Autodesk Inventor part; units mm, degrees
(part 3 of 3)
sketch "LED Slots Sketch" plane through (-133.332, 2.75, -3) normal (0, 1, 0) x (1, 0, 0)
  line L0 (133.332, -3) -> (0, -3) construction
  line L1 (116.6655, -31.8672) -> (16.6665, -31.8672) construction
  line L2 (83.3325, -89.6017) -> (49.9995, -89.6017) construction
  line L3 (116.6655, -31.8672) -> (116.6655, -3) construction
  line L4 (99.999, -60.7344) -> (33.333, -60.7344) construction
  line L5 (99.999, -60.7344) -> (99.999, -31.8672) construction
  line L6 (83.3325, -89.6017) -> (83.3325, -60.7344) construction
  line L7 (66.666, -118.4689) -> (66.666, -89.6017) construction
  line L8 (49.9995, -89.6017) -> (49.9995, -3) construction
  line L9 (16.6665, -31.8672) -> (16.6665, -3) construction
  line L10 (33.333, -60.7344) -> (33.333, -3) construction
  line L11 (66.666, -89.6017) -> (66.666, -3) construction
  line L12 (83.3325, -60.7344) -> (83.3325, -3) construction
  line L13 (99.999, -31.8672) -> (99.999, -3) construction
  line L14 (102.499, -19.9336) -> (97.499, -19.9336) construction
  line L15 (97.499, -19.9336) -> (97.499, -14.9336) construction
  line L16 (97.499, -14.9336) -> (102.499, -14.9336) construction
  line L17 (102.499, -14.9336) -> (102.499, -19.9336) construction
  line L18 (99.999, -22.5586) -> (99.999, -12.3086) construction
  line L19 (108.3322, -17.4336) -> (91.6657, -17.4336) construction
  line L20 (96.999, -20.4336) -> (94.499, -20.4336) construction
  line L21 (94.499, -20.4336) -> (94.499, -14.4336) construction
  line L22 (94.499, -14.4336) -> (96.999, -14.4336) construction
  line L23 (96.999, -14.4336) -> (96.999, -20.4336) construction
  line L24 (108.3322, -22.5586) -> (91.6657, -22.5586) construction
  line L25 (91.6657, -22.5586) -> (91.6657, -12.3086) construction
  line L26 (91.6657, -12.3086) -> (108.3322, -12.3086) construction
  line L27 (108.3322, -12.3086) -> (108.3322, -22.5586) construction
  line L28 (104.499, -12.3086) -> (104.499, -22.5586) construction
  line L29 (92.499, -12.3086) -> (92.499, -22.5586) construction
  line L30 (85.8325, -19.9336) -> (80.8325, -19.9336) construction
  line L31 (80.8325, -19.9336) -> (80.8325, -14.9336) construction
  line L32 (80.8325, -14.9336) -> (85.8325, -14.9336) construction
  line L33 (85.8325, -14.9336) -> (85.8325, -19.9336) construction
  line L34 (83.3325, -22.5586) -> (83.3325, -12.3086) construction
  line L35 (91.6657, -17.4336) -> (74.9992, -17.4336) construction
  line L36 (80.3325, -20.4336) -> (77.8325, -20.4336) construction
  line L37 (77.8325, -20.4336) -> (77.8325, -14.4336) construction
  line L38 (77.8325, -14.4336) -> (80.3325, -14.4336) construction
  line L39 (80.3325, -14.4336) -> (80.3325, -20.4336) construction
  line L40 (91.6657, -22.5586) -> (74.9992, -22.5586) construction
  line L41 (74.9992, -22.5586) -> (74.9992, -12.3086) construction
  line L42 (74.9992, -12.3086) -> (91.6657, -12.3086) construction
  line L43 (91.6657, -12.3086) -> (91.6657, -22.5586) construction
  line L44 (87.8325, -12.3086) -> (87.8325, -22.5586) construction
  line L45 (75.8325, -12.3086) -> (75.8325, -22.5586) construction
  line L46 (69.166, -19.9336) -> (64.166, -19.9336) construction
  line L47 (64.166, -19.9336) -> (64.166, -14.9336) construction
  line L48 (64.166, -14.9336) -> (69.166, -14.9336) construction
  line L49 (69.166, -14.9336) -> (69.166, -19.9336) construction
  line L50 (66.666, -22.5586) -> (66.666, -12.3086) construction
  line L51 (74.9992, -17.4336) -> (58.3327, -17.4336) construction
  line L52 (63.666, -20.4336) -> (61.166, -20.4336) construction
  line L53 (61.166, -20.4336) -> (61.166, -14.4336) construction
  line L54 (61.166, -14.4336) -> (63.666, -14.4336) construction
  line L55 (63.666, -14.4336) -> (63.666, -20.4336) construction
  line L56 (74.9992, -22.5586) -> (58.3327, -22.5586) construction
  line L57 (58.3327, -22.5586) -> (58.3327, -12.3086) construction
  line L58 (58.3327, -12.3086) -> (74.9992, -12.3086) construction
  line L59 (74.9992, -12.3086) -> (74.9992, -22.5586) construction
  line L60 (71.166, -12.3086) -> (71.166, -22.5586) construction
  line L61 (59.166, -12.3086) -> (59.166, -22.5586) construction
  line L62 (35.833, -19.9336) -> (30.833, -19.9336) construction
  line L63 (30.833, -19.9336) -> (30.833, -14.9336) construction
  line L64 (30.833, -14.9336) -> (35.833, -14.9336) construction
  line L65 (35.833, -14.9336) -> (35.833, -19.9336) construction
  line L66 (33.333, -22.5586) -> (33.333, -12.3086) construction
  line L67 (41.6662, -17.4336) -> (24.9997, -17.4336) construction
  line L68 (30.333, -20.4336) -> (27.833, -20.4336) construction
  line L69 (27.833, -20.4336) -> (27.833, -14.4336) construction
  line L70 (27.833, -14.4336) -> (30.333, -14.4336) construction
  line L71 (30.333, -14.4336) -> (30.333, -20.4336) construction
  line L72 (41.6662, -22.5586) -> (24.9997, -22.5586) construction
  line L73 (24.9997, -22.5586) -> (24.9997, -12.3086) construction
  line L74 (24.9997, -12.3086) -> (41.6662, -12.3086) construction
  line L75 (41.6662, -12.3086) -> (41.6662, -22.5586) construction
  line L76 (37.833, -12.3086) -> (37.833, -22.5586) construction
  line L77 (25.833, -12.3086) -> (25.833, -22.5586) construction
  line L78 (52.4995, -19.9336) -> (47.4995, -19.9336) construction
  line L79 (47.4995, -19.9336) -> (47.4995, -14.9336) construction
  line L80 (47.4995, -14.9336) -> (52.4995, -14.9336) construction
  line L81 (52.4995, -14.9336) -> (52.4995, -19.9336) construction
  line L82 (49.9995, -22.5586) -> (49.9995, -12.3086) construction
  line L83 (58.3327, -17.4336) -> (41.6662, -17.4336) construction
  line L84 (46.9995, -20.4336) -> (44.4995, -20.4336) construction
  line L85 (44.4995, -20.4336) -> (44.4995, -14.4336) construction
  line L86 (44.4995, -14.4336) -> (46.9995, -14.4336) construction
  line L87 (46.9995, -14.4336) -> (46.9995, -20.4336) construction
  line L88 (58.3327, -22.5586) -> (41.6662, -22.5586) construction
  line L89 (41.6662, -22.5586) -> (41.6662, -12.3086) construction
  line L90 (41.6662, -12.3086) -> (58.3327, -12.3086) construction
  line L91 (58.3327, -12.3086) -> (58.3327, -22.5586) construction
  line L92 (54.4995, -12.3086) -> (54.4995, -22.5586) construction
  line L93 (42.4995, -12.3086) -> (42.4995, -22.5586) construction
  line L94 (19.1665, -19.9336) -> (14.1665, -19.9336) construction
  line L95 (14.1665, -19.9336) -> (14.1665, -14.9336) construction
  line L96 (14.1665, -14.9336) -> (19.1665, -14.9336) construction
  line L97 (19.1665, -14.9336) -> (19.1665, -19.9336) construction
  line L98 (16.6665, -22.5586) -> (16.6665, -12.3086) construction
  line L99 (24.9997, -17.4336) -> (8.3332, -17.4336) construction
  line L100 (13.6665, -20.4336) -> (11.1665, -20.4336) construction
  line L101 (11.1665, -20.4336) -> (11.1665, -14.4336) construction
  line L102 (11.1665, -14.4336) -> (13.6665, -14.4336) construction
  line L103 (13.6665, -14.4336) -> (13.6665, -20.4336) construction
  line L104 (24.9997, -22.5586) -> (8.3332, -22.5586) construction
  line L105 (8.3332, -22.5586) -> (8.3332, -12.3086) construction
  line L106 (8.3332, -12.3086) -> (24.9997, -12.3086) construction
  line L107 (24.9997, -12.3086) -> (24.9997, -22.5586) construction
  line L108 (21.1665, -12.3086) -> (21.1665, -22.5586) construction
  line L109 (9.1665, -12.3086) -> (9.1665, -22.5586) construction
  line L110 (69.166, -77.6681) -> (64.166, -77.6681) construction
  line L111 (64.166, -77.6681) -> (64.166, -72.6681) construction
  line L112 (64.166, -72.6681) -> (69.166, -72.6681) construction
  line L113 (69.166, -72.6681) -> (69.166, -77.6681) construction
  line L114 (66.666, -80.2931) -> (66.666, -70.0431) construction
  line L115 (74.9992, -75.1681) -> (58.3327, -75.1681) construction
  line L116 (63.666, -78.1681) -> (61.166, -78.1681) construction
  line L117 (61.166, -78.1681) -> (61.166, -72.1681) construction
  line L118 (61.166, -72.1681) -> (63.666, -72.1681) construction
  line L119 (63.666, -72.1681) -> (63.666, -78.1681) construction
  line L120 (74.9992, -80.2931) -> (58.3327, -80.2931) construction
  line L121 (58.3327, -80.2931) -> (58.3327, -70.0431) construction
  line L122 (58.3327, -70.0431) -> (74.9992, -70.0431) construction
  line L123 (74.9992, -70.0431) -> (74.9992, -80.2931) construction
  line L124 (71.166, -70.0431) -> (71.166, -80.2931) construction
  line L125 (59.166, -70.0431) -> (59.166, -80.2931) construction
  line L126 (52.4995, -77.6681) -> (47.4995, -77.6681) construction
  line L127 (47.4995, -77.6681) -> (47.4995, -72.6681) construction
  line L128 (47.4995, -72.6681) -> (52.4995, -72.6681) construction
  line L129 (52.4995, -72.6681) -> (52.4995, -77.6681) construction
  line L130 (49.9995, -80.2931) -> (49.9995, -70.0431) construction
  line L131 (58.3327, -75.1681) -> (41.6662, -75.1681) construction
  line L132 (46.9995, -78.1681) -> (44.4995, -78.1681) construction
  line L133 (44.4995, -78.1681) -> (44.4995, -72.1681) construction
  line L134 (44.4995, -72.1681) -> (46.9995, -72.1681) construction
  line L135 (46.9995, -72.1681) -> (46.9995, -78.1681) construction
  line L136 (58.3327, -80.2931) -> (41.6662, -80.2931) construction
  line L137 (41.6662, -80.2931) -> (41.6662, -70.0431) construction
  line L138 (41.6662, -70.0431) -> (58.3327, -70.0431) construction
  line L139 (58.3327, -70.0431) -> (58.3327, -80.2931) construction
  line L140 (54.4995, -70.0431) -> (54.4995, -80.2931) construction
  line L141 (42.4995, -70.0431) -> (42.4995, -80.2931) construction
  line L142 (30.833, -43.8008) -> (35.833, -43.8008) construction
  line L143 (35.833, -43.8008) -> (35.833, -48.8008) construction
  line L144 (35.833, -48.8008) -> (30.833, -48.8008) construction
  line L145 (30.833, -48.8008) -> (30.833, -43.8008) construction
  line L146 (33.333, -41.1758) -> (33.333, -51.4258) construction
  line L147 (24.9997, -46.3008) -> (41.6662, -46.3008) construction
  line L148 (36.333, -43.3008) -> (38.833, -43.3008) construction
  line L149 (38.833, -43.3008) -> (38.833, -49.3008) construction
  line L150 (38.833, -49.3008) -> (36.333, -49.3008) construction
  line L151 (36.333, -49.3008) -> (36.333, -43.3008) construction
  line L152 (24.9997, -41.1758) -> (41.6662, -41.1758) construction
  line L153 (41.6662, -41.1758) -> (41.6662, -51.4258) construction
  line L154 (41.6662, -51.4258) -> (24.9997, -51.4258) construction
  line L155 (24.9997, -51.4258) -> (24.9997, -41.1758) construction
  line L156 (28.833, -51.4258) -> (28.833, -41.1758) construction
  line L157 (40.833, -51.4258) -> (40.833, -41.1758) construction
  line L158 (85.8325, -77.6681) -> (80.8325, -77.6681) construction
  line L159 (80.8325, -77.6681) -> (80.8325, -72.6681) construction
  line L160 (80.8325, -72.6681) -> (85.8325, -72.6681) construction
  line L161 (85.8325, -72.6681) -> (85.8325, -77.6681) construction
  line L162 (83.3325, -80.2931) -> (83.3325, -70.0431) construction
  line L163 (91.6657, -75.1681) -> (74.9992, -75.1681) construction
  line L164 (80.3325, -78.1681) -> (77.8325, -78.1681) construction
  line L165 (77.8325, -78.1681) -> (77.8325, -72.1681) construction
  line L166 (77.8325, -72.1681) -> (80.3325, -72.1681) construction
  line L167 (80.3325, -72.1681) -> (80.3325, -78.1681) construction
  line L168 (91.6657, -80.2931) -> (74.9992, -80.2931) construction
  line L169 (74.9992, -80.2931) -> (74.9992, -70.0431) construction
  line L170 (74.9992, -70.0431) -> (91.6657, -70.0431) construction
  line L171 (91.6657, -70.0431) -> (91.6657, -80.2931) construction
  line L172 (87.8325, -70.0431) -> (87.8325, -80.2931) construction
  line L173 (75.8325, -70.0431) -> (75.8325, -80.2931) construction
  line L174 (64.166, -43.8008) -> (69.166, -43.8008) construction
  line L175 (69.166, -43.8008) -> (69.166, -48.8008) construction
  line L176 (69.166, -48.8008) -> (64.166, -48.8008) construction
  line L177 (64.166, -48.8008) -> (64.166, -43.8008) construction
  line L178 (66.666, -41.1758) -> (66.666, -51.4258) construction
  line L179 (58.3327, -46.3008) -> (74.9992, -46.3008) construction
  line L180 (69.666, -43.3008) -> (72.166, -43.3008) construction
  line L181 (72.166, -43.3008) -> (72.166, -49.3008) construction
  line L182 (72.166, -49.3008) -> (69.666, -49.3008) construction
  line L183 (69.666, -49.3008) -> (69.666, -43.3008) construction
  line L184 (58.3327, -41.1758) -> (74.9992, -41.1758) construction
  line L185 (74.9992, -41.1758) -> (74.9992, -51.4258) construction
  line L186 (74.9992, -51.4258) -> (58.3327, -51.4258) construction
  line L187 (58.3327, -51.4258) -> (58.3327, -41.1758) construction
  line L188 (62.166, -51.4258) -> (62.166, -41.1758) construction
  line L189 (74.166, -51.4258) -> (74.166, -41.1758) construction
  line L190 (80.8325, -43.8008) -> (85.8325, -43.8008) construction
  line L191 (85.8325, -43.8008) -> (85.8325, -48.8008) construction
  line L192 (85.8325, -48.8008) -> (80.8325, -48.8008) construction
  line L193 (80.8325, -48.8008) -> (80.8325, -43.8008) construction
  line L194 (83.3325, -41.1758) -> (83.3325, -51.4258) construction
  line L195 (74.9992, -46.3008) -> (91.6657, -46.3008) construction
  line L196 (86.3325, -43.3008) -> (88.8325, -43.3008) construction
  line L197 (88.8325, -43.3008) -> (88.8325, -49.3008) construction
  line L198 (88.8325, -49.3008) -> (86.3325, -49.3008) construction
  line L199 (86.3325, -49.3008) -> (86.3325, -43.3008) construction
  line L200 (74.9992, -41.1758) -> (91.6657, -41.1758) construction
  line L201 (91.6657, -41.1758) -> (91.6657, -51.4258) construction
  line L202 (91.6657, -51.4258) -> (74.9992, -51.4258) construction
  line L203 (74.9992, -51.4258) -> (74.9992, -41.1758) construction
  line L204 (78.8325, -51.4258) -> (78.8325, -41.1758) construction
  line L205 (90.8325, -51.4258) -> (90.8325, -41.1758) construction
  line L206 (47.4995, -43.8008) -> (52.4995, -43.8008) construction
  line L207 (52.4995, -43.8008) -> (52.4995, -48.8008) construction
  line L208 (52.4995, -48.8008) -> (47.4995, -48.8008) construction
  line L209 (47.4995, -48.8008) -> (47.4995, -43.8008) construction
  line L210 (49.9995, -41.1758) -> (49.9995, -51.4258) construction
  line L211 (41.6662, -46.3008) -> (58.3327, -46.3008) construction
  line L212 (52.9995, -43.3008) -> (55.4995, -43.3008) construction
  line L213 (55.4995, -43.3008) -> (55.4995, -49.3008) construction
  line L214 (55.4995, -49.3008) -> (52.9995, -49.3008) construction
  line L215 (52.9995, -49.3008) -> (52.9995, -43.3008) construction
  line L216 (41.6662, -41.1758) -> (58.3327, -41.1758) construction
  line L217 (58.3327, -41.1758) -> (58.3327, -51.4258) construction
  line L218 (58.3327, -51.4258) -> (41.6662, -51.4258) construction
  line L219 (41.6662, -51.4258) -> (41.6662, -41.1758) construction
  line L220 (45.4995, -51.4258) -> (45.4995, -41.1758) construction
  line L221 (57.4995, -51.4258) -> (57.4995, -41.1758) construction
  line L222 (97.499, -43.8008) -> (102.499, -43.8008) construction
  line L223 (102.499, -43.8008) -> (102.499, -48.8008) construction
  line L224 (102.499, -48.8008) -> (97.499, -48.8008) construction
  line L225 (97.499, -48.8008) -> (97.499, -43.8008) construction
  line L226 (99.999, -41.1758) -> (99.999, -51.4258) construction
  line L227 (91.6657, -46.3008) -> (108.3322, -46.3008) construction
  line L228 (102.999, -43.3008) -> (105.499, -43.3008) construction
  line L229 (105.499, -43.3008) -> (105.499, -49.3008) construction
  line L230 (105.499, -49.3008) -> (102.999, -49.3008) construction
  line L231 (102.999, -49.3008) -> (102.999, -43.3008) construction
  line L232 (91.6657, -41.1758) -> (108.3322, -41.1758) construction
  line L233 (108.3322, -41.1758) -> (108.3322, -51.4258) construction
  line L234 (108.3322, -51.4258) -> (91.6657, -51.4258) construction
  line L235 (91.6657, -51.4258) -> (91.6657, -41.1758) construction
  line L236 (95.499, -51.4258) -> (95.499, -41.1758) construction
  line L237 (107.499, -51.4258) -> (107.499, -41.1758) construction
  line L238 (64.166, -101.5353) -> (69.166, -101.5353) construction
  line L239 (69.166, -101.5353) -> (69.166, -106.5353) construction
  line L240 (69.166, -106.5353) -> (64.166, -106.5353) construction
  line L241 (64.166, -106.5353) -> (64.166, -101.5353) construction
  line L242 (66.666, -98.9103) -> (66.666, -109.1603) construction
  line L243 (58.3327, -104.0353) -> (74.9992, -104.0353) construction
  line L244 (69.666, -101.0353) -> (72.166, -101.0353) construction
  line L245 (72.166, -101.0353) -> (72.166, -107.0353) construction
  line L246 (72.166, -107.0353) -> (69.666, -107.0353) construction
  line L247 (69.666, -107.0353) -> (69.666, -101.0353) construction
  line L248 (58.3327, -98.9103) -> (74.9992, -98.9103) construction
  line L249 (74.9992, -98.9103) -> (74.9992, -109.1603) construction
  line L250 (74.9992, -109.1603) -> (58.3327, -109.1603) construction
  line L251 (58.3327, -109.1603) -> (58.3327, -98.9103) construction
  line L252 (62.166, -109.1603) -> (62.166, -98.9103) construction
  line L253 (74.166, -109.1603) -> (74.166, -98.9103) construction
  line L254 (119.1655, -19.9336) -> (114.1655, -19.9336) construction
  line L255 (114.1655, -19.9336) -> (114.1655, -14.9336) construction
  line L256 (114.1655, -14.9336) -> (119.1655, -14.9336) construction
  line L257 (119.1655, -14.9336) -> (119.1655, -19.9336) construction
  line L258 (116.6655, -22.5586) -> (116.6655, -12.3086) construction
  line L259 (124.9987, -17.4336) -> (108.3322, -17.4336) construction
  line L260 (113.6655, -20.4336) -> (111.1655, -20.4336) construction
  line L261 (111.1655, -20.4336) -> (111.1655, -14.4336) construction
  line L262 (111.1655, -14.4336) -> (113.6655, -14.4336) construction
  line L263 (113.6655, -14.4336) -> (113.6655, -20.4336) construction
  line L264 (124.9987, -22.5586) -> (108.3322, -22.5586) construction
  line L265 (108.3322, -22.5586) -> (108.3322, -12.3086) construction
  line L266 (108.3322, -12.3086) -> (124.9987, -12.3086) construction
  line L267 (124.9987, -12.3086) -> (124.9987, -22.5586) construction
  line L268 (121.1655, -12.3086) -> (121.1655, -22.5586) construction
  line L269 (109.1655, -12.3086) -> (109.1655, -22.5586) construction
  line L270 (119.1655, -22.5586) -> (119.1655, -12.3086) projected
  line L271 (121.1655, -22.5586) -> (121.1655, -12.3086) projected
  arc A0 (119.1655, -22.5586) -> (121.1655, -22.5586) centre (120.1655, -22.5586) ccw projected
  arc A1 (121.1655, -12.3086) -> (119.1655, -12.3086) centre (120.1655, -12.3086) ccw projected
  line L272 (9.1665, -22.5586) -> (9.1665, -12.3086) projected
  line L273 (11.1665, -22.5586) -> (11.1665, -12.3086) projected
  arc A2 (9.1665, -22.5586) -> (11.1665, -22.5586) centre (10.1665, -22.5586) ccw projected
  arc A3 (11.1665, -12.3086) -> (9.1665, -12.3086) centre (10.1665, -12.3086) ccw projected
  line L274 (28.833, -51.4258) -> (28.833, -41.1758) projected
  line L275 (30.833, -51.4258) -> (30.833, -41.1758) projected
  arc A4 (28.833, -51.4258) -> (30.833, -51.4258) centre (29.833, -51.4258) ccw projected
  arc A5 (30.833, -41.1758) -> (28.833, -41.1758) centre (29.833, -41.1758) ccw projected
  line L276 (105.499, -51.4258) -> (105.499, -41.1758) projected
  line L277 (107.499, -51.4258) -> (107.499, -41.1758) projected
  arc A6 (105.499, -51.4258) -> (107.499, -51.4258) centre (106.499, -51.4258) ccw projected
  arc A7 (107.499, -41.1758) -> (105.499, -41.1758) centre (106.499, -41.1758) ccw projected
  line L278 (42.4995, -80.2931) -> (42.4995, -70.0431) projected
  line L279 (44.4995, -80.2931) -> (44.4995, -70.0431) projected
  arc A8 (42.4995, -80.2931) -> (44.4995, -80.2931) centre (43.4995, -80.2931) ccw projected
  arc A9 (44.4995, -70.0431) -> (42.4995, -70.0431) centre (43.4995, -70.0431) ccw projected
  line L280 (85.8325, -80.2931) -> (85.8325, -70.0431) projected
  line L281 (87.8325, -80.2931) -> (87.8325, -70.0431) projected
  arc A10 (85.8325, -80.2931) -> (87.8325, -80.2931) centre (86.8325, -80.2931) ccw projected
  arc A11 (87.8325, -70.0431) -> (85.8325, -70.0431) centre (86.8325, -70.0431) ccw projected
  line L282 (72.166, -109.1603) -> (72.166, -98.9103) projected
  line L283 (74.166, -109.1603) -> (74.166, -98.9103) projected
  arc A12 (72.166, -109.1603) -> (74.166, -109.1603) centre (73.166, -109.1603) ccw projected
  arc A13 (74.166, -98.9103) -> (72.166, -98.9103) centre (73.166, -98.9103) ccw projected
  line L284 (62.166, -109.1603) -> (62.166, -98.9103) projected
  line L285 (64.166, -109.1603) -> (64.166, -98.9103) projected
  arc A14 (62.166, -109.1603) -> (64.166, -109.1603) centre (63.166, -109.1603) ccw projected
  arc A15 (64.166, -98.9103) -> (62.166, -98.9103) centre (63.166, -98.9103) ccw projected
  point P0 (119.1655, -17.4336)
  point P1 (11.1665, -17.4336)
  point P2 (11.1665, -17.4336)
  point P3 (72.166, -104.0353)
  point P4 (72.166, -104.0353)
  point P5 (64.166, -104.0353)
  point P6 (85.8325, -75.1681)
  point P7 (64.166, -104.0353)
  point P8 (105.499, -46.3008)
  point P9 (105.499, -46.3008)
  point P10 (44.4995, -75.1681)
  point P11 (44.4995, -75.1681)
  point P12 (30.833, -46.3008)
  constraints: 4 coincident, 17 other
derived "g16-ledframe.ipt"
extrude "Extrusion2" cut sketch "LED Slots Sketch" against normal through all
equation "\"d6\" = LayerThickness"
equation "\"d8\" = Bolt_HoleDiameter"
equation "\"LayerThickness\" = 2.75"
equation "\"Bolt_HoleDiameter\" = 3"
body "Solid2"
